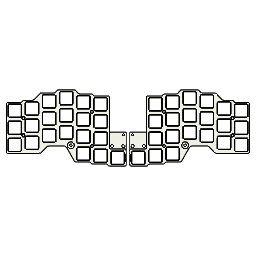
mriya-top-plate-v1.02 (Autodesk Fusion 360 design; units mm, degrees)
Autodesk Fusion 360 part; units mm, degrees
note: some values were not read from the file. Set by a fixed rule: which sketch regions a step uses.
sketch "mriya-top-plate" plane through (0, 0, 0) normal (0, 0, 1) x (1, 0, 0)
  arc A0 (-117.8, 77.3932) -> (-119.9, 79.4932) centre (-119.9, 77.3932) ccw
  line L0 (-132.4, 59.0932) -> (-132.4, 46.6932)
  line L1 (-114, 60.4932) -> (-114, 49.6932)
  arc A1 (-131.6, 78.8932) -> (-132.4, 78.0932) centre (-131.6, 78.0932) ccw
  line L2 (-131.6, 59.8932) -> (-119.2, 59.8932)
  circle A2 centre (-115.9, 63.5432) radius 1.45
  line L3 (-117.8, 58.3932) -> (-117.8, 47.5932)
  line L4 (-130.9, 60.4932) -> (-119.9, 60.4932)
  arc A3 (-131.6, 59.8932) -> (-132.4, 59.0932) centre (-131.6, 59.0932) ccw
  line L5 (-130.9, 79.4932) -> (-119.9, 79.4932)
  arc A4 (-119.2, 64.8932) -> (-118.4, 65.6932) centre (-119.2, 65.6932) ccw
  line L6 (-130.9, 64.2932) -> (-120.1, 64.2932)
  line L7 (-134.6, 79.4932) -> (-134.6, 26.2932) construction
  line L8 (-133, 77.3932) -> (-133, 66.3932)
  line L9 (-133.1, 81.1432) -> (-119.0284, 81.1432)
  line L10 (-117.8, 77.3932) -> (-117.8, 66.5932)
  line L11 (-131.6, 78.8932) -> (-119.2, 78.8932)
  arc A5 (-115.0716, 83.4432) -> (-116.5919, 82.8135) centre (-115.0716, 81.2933) ccw
  line L12 (-106.1426, 83.2932) -> (-115.0716, 83.2932) construction
  arc A6 (-115.0716, 83.2932) -> (-116.4858, 82.7074) centre (-115.0716, 81.2933) ccw construction
  arc A7 (-119.0284, 80.9932) -> (-117.6142, 81.579) centre (-119.0284, 82.9932) ccw construction
  arc A8 (-118.4, 59.0932) -> (-119.2, 59.8932) centre (-119.2, 59.0932) ccw
  arc A9 (-133, 66.3932) -> (-130.9, 64.2932) centre (-130.9, 66.3932) ccw
  line L13 (-133, 58.3932) -> (-133, 47.3932)
  line L14 (-113.4, 61.3932) -> (-113.4, 48.9932)
  arc A10 (-133.1, 80.9932) -> (-134.6, 79.4932) centre (-133.1, 79.4932) ccw construction
  arc A11 (-133.1, 81.1432) -> (-134.75, 79.4932) centre (-133.1, 79.4932) ccw
  line L15 (-74.6, 40.6932) -> (-62.2, 40.6932)
  line L16 (-73.9, 40.0932) -> (-62.9, 40.0932)
  line L17 (-73.9, 78.0932) -> (-62.9, 78.0932)
  arc A12 (-134.6, 26.2932) -> (-133.1, 24.7932) centre (-133.1, 26.2932) ccw construction
  arc A13 (-131.6, 40.8932) -> (-132.4, 40.0932) centre (-131.6, 40.0932) ccw
  arc A14 (-130.9, 41.4932) -> (-133, 39.3932) centre (-130.9, 39.3932) ccw
  arc A15 (-119.2, 26.8932) -> (-118.4, 27.6932) centre (-119.2, 27.6932) ccw
  line L18 (-73.9, 55.2932) -> (-62.9, 55.2932)
  line L19 (-74.6, 54.6932) -> (-62.2, 54.6932)
  arc A16 (-114, 30.6932) -> (-111.9, 28.5932) centre (-111.9, 30.6932) ccw
  line L20 (-113.4, 42.3932) -> (-113.4, 29.9932)
  line L21 (-130.9, 26.2932) -> (-119.9, 26.2932)
  line L22 (-59.6047, 16.0356) -> (-67.8823, 30.687)
  arc A17 (-119.9, 26.2932) -> (-117.8, 28.3932) centre (-119.9, 28.3932) ccw
  line L23 (-74.6, 92.6932) -> (-62.2, 92.6932)
  line L24 (-132.4, 40.0932) -> (-132.4, 27.6932)
  arc A18 (-113.4, 29.9932) -> (-112.6, 29.1932) centre (-112.6, 29.9932) ccw
  line L25 (-130.9, 41.4932) -> (-119.9, 41.4932)
  arc A19 (-118.4, 40.0932) -> (-119.2, 40.8932) centre (-119.2, 40.0932) ccw
  line L26 (-77.0716, 94.7932) -> (-59.7284, 94.7932) construction
  line L27 (-114, 41.4932) -> (-114, 30.6932)
  arc A20 (-132.4, 27.6932) -> (-131.6, 26.8932) centre (-131.6, 27.6932) ccw
  arc A21 (-133, 28.3932) -> (-130.9, 26.2932) centre (-130.9, 28.3932) ccw
  line L28 (-117.8, 39.3932) -> (-117.8, 28.3932)
  line L29 (-131.6, 40.8932) -> (-119.2, 40.8932)
  line L30 (-73.9, 59.0932) -> (-62.9, 59.0932)
  arc A22 (-117.8, 39.3932) -> (-119.9, 41.4932) centre (-119.9, 39.3932) ccw
  line L31 (-131.6, 26.8932) -> (-119.2, 26.8932)
  line L32 (-74.6, 78.6932) -> (-62.2, 78.6932)
  line L33 (-112.6, 29.1932) -> (-100.2, 29.1932)
  line L34 (-111.9, 66.5932) -> (-100.9, 66.5932)
  line L35 (-130.9, 45.2932) -> (-120.1, 45.2932)
  arc A23 (-133, 47.3932) -> (-130.9, 45.2932) centre (-130.9, 47.3932) ccw
  line L36 (-112.6, 62.1932) -> (-100.2, 62.1932)
  arc A24 (-120.1, 45.2932) -> (-117.8, 47.5932) centre (-120.1, 47.5932) ccw
  arc A25 (-119.2, 45.8932) -> (-118.4, 46.6932) centre (-119.2, 46.6932) ccw
  line L37 (-133.1, 24.7932) -> (-98.1426, 24.7932) construction
  line L38 (-131.6, 45.8932) -> (-119.2, 45.8932)
  arc A26 (-132.4, 46.6932) -> (-131.6, 45.8932) centre (-131.6, 46.6932) ccw
  line L39 (-111.7, 62.7932) -> (-100.9, 62.7932)
  line L40 (-104.1274, 84.2779) -> (-97.5918, 90.8135)
  circle A27 centre (-63.3, 33.4932) radius 1.4
  arc A28 (-114, 49.6932) -> (-111.9, 47.5932) centre (-111.9, 49.6932) ccw
  line L41 (-111.9, 47.5932) -> (-100.9, 47.5932)
  arc A29 (-111.7, 43.7932) -> (-114, 41.4932) centre (-111.7, 41.4932) ccw
  circle A30 centre (-63.3, 33.4932) radius 3.8
  line L42 (-133.1, 24.6432) -> (-98.1426, 24.6432)
  line L43 (-133, 39.3932) -> (-133, 28.3932)
  line L44 (-74.6, 73.6932) -> (-62.2, 73.6932)
  line L45 (-118.4, 40.0932) -> (-118.4, 27.6932)
  arc A31 (-113.4, 48.9932) -> (-112.6, 48.1932) centre (-112.6, 48.9932) ccw
  circle A32 centre (-115.9, 44.5432) radius 1.45
  line L46 (-74.6, 59.6932) -> (-62.2, 59.6932)
  line L47 (-112.6, 81.1932) -> (-100.2, 81.1932)
  line L48 (-134.75, 79.4932) -> (-134.75, 26.2932)
  line L49 (-118.4, 59.0932) -> (-118.4, 46.6932)
  line L50 (-111.7, 43.7932) -> (-100.9, 43.7932)
  arc A33 (-113.4, 67.9932) -> (-112.6, 67.1932) centre (-112.6, 67.9932) ccw
  arc A34 (-111.9, 81.7932) -> (-114, 79.6932) centre (-111.9, 79.6932) ccw
  arc A35 (-106.1426, 83.4432) -> (-104.1274, 84.2779) centre (-106.1426, 86.2932) ccw
  line L51 (-111.9, 81.7932) -> (-100.9, 81.7932)
  arc A36 (-114, 68.6932) -> (-111.9, 66.5932) centre (-111.9, 68.6932) ccw
  line L52 (-112.6, 43.1932) -> (-100.2, 43.1932)
  arc A37 (-111.7, 62.7932) -> (-114, 60.4932) centre (-111.7, 60.4932) ccw
  arc A38 (-112.6, 81.1932) -> (-113.4, 80.3932) centre (-112.6, 80.3932) ccw
  arc A39 (-106.1426, 83.2932) -> (-104.0213, 84.1719) centre (-106.1426, 86.2932) ccw construction
  line L53 (-114, 79.6932) -> (-114, 68.6932)
  line L54 (-112.6, 48.1932) -> (-100.2, 48.1932)
  line L55 (-112.6, 67.1932) -> (-100.2, 67.1932)
  line L56 (-111.9, 28.5932) -> (-100.9, 28.5932)
  line L57 (-113.4, 80.3932) -> (-113.4, 67.9932)
  arc A40 (-112.6, 62.1932) -> (-113.4, 61.3932) centre (-112.6, 61.3932) ccw
  line L58 (-106.1426, 83.4432) -> (-115.0716, 83.4432)
  line L59 (-104.0213, 84.1719) -> (-97.4858, 90.7074) construction
  arc A41 (-10.1, 30.7932) -> (-10.1, 34.1932) centre (-10.1, 32.4932) ccw construction
  line L60 (-36.6, 33.8932) -> (-24.2, 33.8932)
  arc A42 (-43.2, 17.1932) -> (-42.4, 17.9932) centre (-43.2, 17.9932) ccw
  line L61 (-36.6, 28.8932) -> (-24.2, 28.8932)
  line L62 (-35.9, 14.2932) -> (-24.9, 14.2932)
  arc A43 (-62.9, 40.0932) -> (-60.8, 42.1932) centre (-62.9, 42.1932) ccw
  line L63 (-55.6, 31.1932) -> (-43.2, 31.1932)
  arc A44 (-43.9, 35.5932) -> (-41.8, 37.6932) centre (-43.9, 37.6932) ccw
  arc A45 (-41.7203, 14.4013) -> (-43.0284, 14.9432) centre (-43.0284, 13.0933) ccw
  line L64 (-35.7, 33.2932) -> (-24.9, 33.2932)
  arc A46 (-56.4, 17.9932) -> (-55.6, 17.1932) centre (-55.6, 17.9932) ccw
  line L65 (-54.9, 16.5932) -> (-43.9, 16.5932)
  line L66 (-39.0716, 12.6432) -> (-24.0284, 12.6432)
  arc A47 (-43.2, 36.1932) -> (-42.4, 36.9932) centre (-43.2, 36.9932) ccw
  arc A48 (-41.8, 29.4932) -> (-44.1, 31.7932) centre (-44.1, 29.4932) ccw
  arc A49 (-41.6142, 14.5074) -> (-43.0284, 15.0932) centre (-43.0284, 13.0933) ccw construction
  arc A50 (-43.9, 16.5932) -> (-41.8, 18.6932) centre (-43.9, 18.6932) ccw
  arc A51 (-42.4, 30.3932) -> (-43.2, 31.1932) centre (-43.2, 30.3932) ccw
  line L67 (-35.9, 29.4932) -> (-24.9, 29.4932)
  line L68 (-36.6, 14.8932) -> (-24.2, 14.8932)
  line L69 (-21.4858, 11.079) -> (-22.6142, 12.2074) construction
  arc A52 (-4.4, 25.7932) -> (-5.2, 26.5932) centre (-5.2, 25.7932) ccw
  line L70 (-18.4, 25.7932) -> (-18.4, 13.3932)
  line L71 (-21.5919, 10.9729) -> (-22.7203, 12.1013)
  line L72 (-17.6, 26.5932) -> (-5.2, 26.5932)
  line L73 (-16.9, 27.1932) -> (-5.7, 27.1932)
  line L74 (-4, 25.4932) -> (-4, 13.6932)
  line L75 (-4.4, 25.7932) -> (-4.4, 13.3932)
  arc A53 (-21.5919, 10.9729) -> (-20.0716, 10.3432) centre (-20.0716, 12.4932) ccw
  line L76 (-2.75, 22.8932) -> (-2.75, 16.2932)
  arc A54 (-3.6, 10.3432) -> (-1.95, 11.9932) centre (-3.6, 11.9932) ccw
  arc A55 (-24.9, 14.2932) -> (-22.8, 16.3932) centre (-24.9, 16.3932) ccw
  line L77 (-17.6, 12.5932) -> (-5.2, 12.5932)
  circle A56 centre (-17.6, 32.4932) radius 1.7
  arc A57 (-22.7203, 12.1013) -> (-24.0284, 12.6432) centre (-24.0284, 10.7933) ccw
  line L78 (-19, 25.0932) -> (-19, 14.0932)
  line L79 (-2.1, 11.9932) -> (-2.1, 28.6932) construction
  arc A58 (-17.6, 26.5932) -> (-18.4, 25.7932) centre (-17.6, 25.7932) ccw
  circle A59 centre (-5.1, 45.1932) radius 1.1
  arc A60 (-5.2, 12.5932) -> (-4.4, 13.3932) centre (-5.2, 13.3932) ccw
  arc A61 (-5.7, 11.9932) -> (-4, 13.6932) centre (-5.7, 13.6932) ccw
  arc A62 (-3.6, 10.4932) -> (-2.1, 11.9932) centre (-3.6, 11.9932) ccw construction
  arc A63 (-12.7, 34.1932) -> (-12.7, 30.7932) centre (-12.7, 32.4932) ccw construction
  line L80 (-22.8, 27.3932) -> (-22.8, 16.3932)
  arc A64 (-19, 14.0932) -> (-16.9, 11.9932) centre (-16.9, 14.0932) ccw
  arc A65 (-36.6, 28.8932) -> (-37.4, 28.0932) centre (-36.6, 28.0932) ccw
  arc A66 (-37.4, 15.6932) -> (-36.6, 14.8932) centre (-36.6, 15.6932) ccw
  circle A67 centre (-39.9, 32.5432) radius 1.45
  arc A68 (-21.4858, 11.079) -> (-20.0716, 10.4932) centre (-20.0716, 12.4932) ccw construction
  line L81 (-23.4, 28.0932) -> (-23.4, 15.6932)
  line L82 (-3.6, 10.3432) -> (-20.0716, 10.3432)
  arc A69 (-24.2, 14.8932) -> (-23.4, 15.6932) centre (-24.2, 15.6932) ccw
  arc A70 (-16.9, 27.1932) -> (-19, 25.0932) centre (-16.9, 25.0932) ccw
  line L83 (-16.9, 11.9932) -> (-5.7, 11.9932)
  arc A71 (-23.4, 28.0932) -> (-24.2, 28.8932) centre (-24.2, 28.0932) ccw
  arc A72 (-22.8, 27.3932) -> (-24.9, 29.4932) centre (-24.9, 27.3932) ccw
  arc A73 (-2.1, 28.6932) -> (-2.9, 29.4932) centre (-2.9, 28.6932) ccw construction
  arc A74 (-18.4, 13.3932) -> (-17.6, 12.5932) centre (-17.6, 13.3932) ccw
  arc A75 (-4, 25.4932) -> (-5.7, 27.1932) centre (-5.7, 25.4932) ccw
  line L84 (-3.6, 10.4932) -> (-20.0716, 10.4932) construction
  line L85 (-1.95, 11.9932) -> (-1.95, 34.4932)
  arc A76 (-22.6142, 12.2074) -> (-24.0284, 12.7932) centre (-24.0284, 10.7933) ccw construction
  arc A77 (-22.8, 84.3932) -> (-24.9, 86.4932) centre (-24.9, 84.3932) ccw
  arc A78 (-37.4, 53.6932) -> (-36.6, 52.8932) centre (-36.6, 53.6932) ccw
  arc A79 (-1.95, 47.3932) -> (-2.75, 48.1932) centre (-2.75, 47.3932) ccw
  line L86 (-20.7, 49.1932) -> (-20.7, 87.3432)
  arc A80 (-35.9, 67.4932) -> (-38, 65.3932) centre (-35.9, 65.3932) ccw
  arc A81 (-35.9, 48.4932) -> (-38, 46.3932) centre (-35.9, 46.3932) ccw
  line L87 (-54.9, 50.7932) -> (-43.9, 50.7932)
  line L88 (-22.8, 84.3932) -> (-22.8, 73.3932)
  arc A82 (-60.8, 53.1932) -> (-62.9, 55.2932) centre (-62.9, 53.1932) ccw
  arc A83 (-24.9, 52.2932) -> (-22.8, 54.3932) centre (-24.9, 54.3932) ccw
  arc A84 (-42.4, 49.3932) -> (-43.2, 50.1932) centre (-43.2, 49.3932) ccw
  arc A85 (-41.8, 48.6932) -> (-43.9, 50.7932) centre (-43.9, 48.6932) ccw
  line L89 (-1.95, 29.4932) -> (-20.7, 29.4932)
  line L90 (-12.7, 34.1932) -> (-10.1, 34.1932) construction
  arc A86 (-24.9, 33.2932) -> (-22.8, 35.3932) centre (-24.9, 35.3932) ccw
  line L91 (-10.1, 30.7932) -> (-12.7, 30.7932) construction
  circle A87 centre (-11.4, 32.4932) radius 1.15 construction
  line L92 (-19.7, 29.4932) -> (-2.9, 29.4932) construction
  circle A88 centre (-5.1, 32.4932) radius 1.7
  arc A89 (-24.2, 33.8932) -> (-23.4, 34.6932) centre (-24.2, 34.6932) ccw
  arc A90 (-37.4, 34.6932) -> (-36.6, 33.8932) centre (-36.6, 34.6932) ccw
  arc A91 (-40.4858, 13.379) -> (-39.0716, 12.7932) centre (-39.0716, 14.7932) ccw construction
  arc A92 (-35.9, 29.4932) -> (-38, 27.3932) centre (-35.9, 27.3932) ccw
  arc A93 (-38, 35.5932) -> (-35.7, 33.2932) centre (-35.7, 35.5932) ccw
  arc A94 (-38, 16.3932) -> (-35.9, 14.2932) centre (-35.9, 16.3932) ccw
  line L93 (-37.4, 28.0932) -> (-37.4, 15.6932)
  arc A95 (-58.3142, 94.2074) -> (-59.7284, 94.7932) centre (-59.7284, 92.7932) ccw construction
  line L94 (-61.4, 72.8932) -> (-61.4, 60.4932)
  line L95 (-36.6, 66.8932) -> (-24.2, 66.8932)
  line L96 (-35.7, 71.2932) -> (-24.9, 71.2932)
  arc A96 (-54.8797, 90.9851) -> (-53.5716, 90.4432) centre (-53.5716, 92.2931) ccw
  line L97 (-54.9, 73.5932) -> (-43.9, 73.5932)
  arc A97 (-58.2081, 94.3135) -> (-59.7284, 94.9432) centre (-59.7284, 92.7932) ccw
  line L98 (-54.9, 88.7932) -> (-43.9, 88.7932)
  line L99 (-35.9, 52.2932) -> (-24.9, 52.2932)
  arc A98 (-54.9, 88.7932) -> (-57, 86.6932) centre (-54.9, 86.6932) ccw
  line L100 (-61.4, 91.8932) -> (-61.4, 79.4932)
  line L101 (-58.2081, 94.3135) -> (-54.8797, 90.9851)
  line L102 (-56.4, 87.3932) -> (-56.4, 74.9932)
  arc A99 (-61.4, 91.8932) -> (-62.2, 92.6932) centre (-62.2, 91.8932) ccw
  line L103 (-55.6, 88.1932) -> (-43.2, 88.1932)
  line L104 (-55.6, 74.1932) -> (-43.2, 74.1932)
  line L105 (-60.8, 72.1932) -> (-60.8, 61.1932)
  arc A100 (-57, 75.6932) -> (-54.9, 73.5932) centre (-54.9, 75.6932) ccw
  circle A101 centre (-39.9, 70.5432) radius 1.45
  arc A102 (-54.9858, 90.879) -> (-53.5716, 90.2932) centre (-53.5716, 92.2931) ccw construction
  arc A103 (-38, 73.5932) -> (-35.7, 71.2932) centre (-35.7, 73.5932) ccw
  arc A104 (-62.9, 78.0932) -> (-60.8, 80.1932) centre (-62.9, 80.1932) ccw
  line L106 (-36.7716, 88.1432) -> (-21.5, 88.1432)
  arc A105 (-56.4, 74.9932) -> (-55.6, 74.1932) centre (-55.6, 74.9932) ccw
  line L107 (-53.5716, 90.4432) -> (-40.7284, 90.4432)
  line L108 (-53.5716, 90.2932) -> (-40.7284, 90.2932) construction
  arc A106 (-62.2, 78.6932) -> (-61.4, 79.4932) centre (-62.2, 79.4932) ccw
  line L109 (-57, 86.6932) -> (-57, 75.6932)
  arc A107 (-60.8, 91.1932) -> (-62.9, 93.2932) centre (-62.9, 91.1932) ccw
  arc A108 (-39.3142, 89.7074) -> (-40.7284, 90.2932) centre (-40.7284, 88.2932) ccw construction
  arc A109 (-38.0797, 88.6851) -> (-36.7716, 88.1432) centre (-36.7716, 89.9932) ccw
  line L110 (-37.4, 85.0932) -> (-37.4, 72.6932)
  arc A110 (-55.6, 88.1932) -> (-56.4, 87.3932) centre (-55.6, 87.3932) ccw
  arc A111 (-60.8, 72.1932) -> (-62.9, 74.2932) centre (-62.9, 72.1932) ccw
  arc A112 (-61.4, 72.8932) -> (-62.2, 73.6932) centre (-62.2, 72.8932) ccw
  line L111 (-60.8, 91.1932) -> (-60.8, 80.1932)
  line L112 (-38.0797, 88.6851) -> (-39.2081, 89.8135)
  line L113 (-58.3142, 94.2074) -> (-54.9858, 90.879) construction
  line L114 (-38.1858, 88.579) -> (-39.3142, 89.7074) construction
  line L115 (-99.4, 42.3932) -> (-99.4, 29.9932)
  arc A113 (-81.2, 37.1932) -> (-80.4, 37.9932) centre (-81.2, 37.9932) ccw
  arc A114 (-75.4, 41.4932) -> (-74.6, 40.6932) centre (-74.6, 41.4932) ccw
  line L116 (-95.9152, 25.5658) -> (-89.6726, 31.8084)
  line L117 (-96.0213, 25.6719) -> (-89.7787, 31.9145) construction
  arc A115 (-76, 42.1932) -> (-73.9, 40.0932) centre (-73.9, 42.1932) ccw
  line L118 (-42.4, 49.3932) -> (-42.4, 36.9932)
  arc A116 (-94.4, 37.9932) -> (-93.6, 37.1932) centre (-93.6, 37.9932) ccw
  arc A117 (-67.7517, 30.7608) -> (-71.2344, 32.7932) centre (-71.2344, 28.793) ccw construction
  arc A118 (-67.8823, 30.687) -> (-71.2344, 32.6432) centre (-71.2344, 28.793) ccw
  line L119 (-98.8, 41.6932) -> (-98.8, 30.6932)
  arc A119 (-98.1426, 24.7932) -> (-96.0213, 25.6719) centre (-98.1426, 27.7931) ccw construction
  arc A120 (-87.6574, 32.7932) -> (-89.7787, 31.9145) centre (-87.6573, 29.7931) ccw construction
  arc A121 (-99.4, 42.3932) -> (-100.2, 43.1932) centre (-100.2, 42.3932) ccw
  arc A122 (-87.6574, 32.6432) -> (-89.6726, 31.8084) centre (-87.6573, 29.7931) ccw
  line L120 (-20.7, 29.4932) -> (-20.7, 49.1932)
  line L121 (-36.6, 52.8932) -> (-24.2, 52.8932)
  line L122 (-57, 48.6932) -> (-57, 37.6932)
  circle A123 centre (-5.1, 45.1932) radius 2.2 construction
  line L123 (-35.9, 86.4932) -> (-24.9, 86.4932)
  line L124 (-1.95, 47.3932) -> (-1.95, 34.4932)
  line L125 (-60.8, 53.1932) -> (-60.8, 42.1932)
  line L126 (-36.7716, 87.9932) -> (-21.5, 87.9932) construction
  line L127 (-23.4, 47.0932) -> (-23.4, 34.6932)
  line L128 (-36.6, 47.8932) -> (-24.2, 47.8932)
  line L129 (-35.9, 48.4932) -> (-24.9, 48.4932)
  line L130 (-36.6, 85.8932) -> (-24.2, 85.8932)
  line L131 (-41.8, 48.6932) -> (-41.8, 37.6932)
  line L132 (-37.4, 47.0932) -> (-37.4, 34.6932)
  line L133 (-36.6, 71.8932) -> (-24.2, 71.8932)
  line L134 (-56.4, 49.3932) -> (-56.4, 36.9932)
  line L135 (-22.8, 46.3932) -> (-22.8, 35.3932)
  line L136 (-38, 46.3932) -> (-38, 35.5932)
  line L137 (-20.7, 30.4932) -> (-20.7, 87.1932) construction
  line L138 (-35.9, 67.4932) -> (-24.9, 67.4932)
  line L139 (-61.4, 53.8932) -> (-61.4, 41.4932)
  line L140 (-95, 68.6932) -> (-95, 57.6932)
  line L141 (-75.4, 72.8932) -> (-75.4, 60.4932)
  line L142 (-79.8, 68.6932) -> (-79.8, 57.6932)
  line L143 (-80.4, 69.3932) -> (-80.4, 56.9932)
  arc A124 (-82.2284, 91.2932) -> (-80.8142, 91.879) centre (-82.2284, 93.2932) ccw construction
  arc A125 (-79.8, 68.6932) -> (-81.9, 70.7932) centre (-81.9, 68.6932) ccw
  line L144 (-76, 72.1932) -> (-76, 61.1932)
  line L145 (-94.4, 69.3932) -> (-94.4, 56.9932)
  arc A126 (-112.6, 43.1932) -> (-113.4, 42.3932) centre (-112.6, 42.3932) ccw
  arc A127 (-134.75, 26.2932) -> (-133.1, 24.6432) centre (-133.1, 26.2932) ccw
  line L146 (-76, 91.1932) -> (-76, 80.1932)
  arc A128 (-73.9, 93.2932) -> (-76, 91.1932) centre (-73.9, 91.1932) ccw
  arc A129 (-77.0716, 94.9432) -> (-78.5919, 94.3135) centre (-77.0716, 92.7933) ccw
  arc A130 (-76, 80.1932) -> (-73.9, 78.0932) centre (-73.9, 80.1932) ccw
  arc A131 (-92.9, 89.7932) -> (-95, 87.6932) centre (-92.9, 87.6932) ccw
  line L147 (-78.4858, 94.2074) -> (-80.8142, 91.879) construction
  arc A132 (-73.9, 74.2932) -> (-76, 72.1932) centre (-73.9, 72.1932) ccw
  arc A133 (-74.6, 73.6932) -> (-75.4, 72.8932) centre (-74.6, 72.8932) ccw
  line L148 (-78.5919, 94.3135) -> (-80.9203, 91.9851)
  line L149 (-79.8, 87.6932) -> (-79.8, 76.6932)
  arc A134 (-75.4, 79.4932) -> (-74.6, 78.6932) centre (-74.6, 79.4932) ccw
  line L150 (-59.4741, 16.1094) -> (-67.7517, 30.7608) construction
  line L151 (-80.4, 88.3932) -> (-80.4, 75.9932)
  line L152 (-75.4, 91.8932) -> (-75.4, 79.4932)
  arc A135 (-77.0716, 94.7932) -> (-78.4858, 94.2074) centre (-77.0716, 92.7933) ccw construction
  arc A136 (-94.4, 75.9932) -> (-93.6, 75.1932) centre (-93.6, 75.9932) ccw
  line L153 (-96.0716, 91.4432) -> (-82.2284, 91.4432)
  arc A137 (-100.2, 67.1932) -> (-99.4, 67.9932) centre (-100.2, 67.9932) ccw
  line L154 (-93.6, 89.1932) -> (-81.2, 89.1932)
  arc A138 (-100.9, 66.5932) -> (-98.8, 68.6932) centre (-100.9, 68.6932) ccw
  arc A139 (-96.0716, 91.2932) -> (-97.4858, 90.7074) centre (-96.0716, 89.2933) ccw construction
  line L155 (-99.4, 80.3932) -> (-99.4, 67.9932)
  arc A140 (-96.0716, 91.4432) -> (-97.5918, 90.8135) centre (-96.0716, 89.2933) ccw
  arc A141 (-92.9, 70.7932) -> (-95, 68.6932) centre (-92.9, 68.6932) ccw
  line L156 (-92.9, 89.7932) -> (-81.9, 89.7932)
  line L157 (-93.6, 70.1932) -> (-81.2, 70.1932)
  line L158 (-95, 87.6932) -> (-95, 76.6932)
  arc A142 (-99.4, 80.3932) -> (-100.2, 81.1932) centre (-100.2, 80.3932) ccw
  line L159 (-92.9, 70.7932) -> (-81.9, 70.7932)
  line L160 (-92.9, 74.5932) -> (-81.9, 74.5932)
  line L161 (-94.4, 88.3932) -> (-94.4, 75.9932)
  line L162 (-93.6, 75.1932) -> (-81.2, 75.1932)
  arc A143 (-93.6, 89.1932) -> (-94.4, 88.3932) centre (-93.6, 88.3932) ccw
  arc A144 (-98.8, 79.6932) -> (-100.9, 81.7932) centre (-100.9, 79.6932) ccw
  arc A145 (-93.6, 70.1932) -> (-94.4, 69.3932) centre (-93.6, 69.3932) ccw
  arc A146 (-80.4, 88.3932) -> (-81.2, 89.1932) centre (-81.2, 88.3932) ccw
  line L163 (-96.0716, 91.2932) -> (-82.2284, 91.2932) construction
  arc A147 (-95, 76.6932) -> (-92.9, 74.5932) centre (-92.9, 76.6932) ccw
  arc A148 (-79.8, 87.6932) -> (-81.9, 89.7932) centre (-81.9, 87.6932) ccw
  arc A149 (-82.2284, 91.4432) -> (-80.9203, 91.9851) centre (-82.2284, 93.2932) ccw
  line L164 (-98.8, 79.6932) -> (-98.8, 68.6932)
  arc A150 (-81.9, 74.5932) -> (-79.8, 76.6932) centre (-81.9, 76.6932) ccw
  arc A151 (-80.4, 69.3932) -> (-81.2, 70.1932) centre (-81.2, 69.3932) ccw
  arc A152 (-81.2, 75.1932) -> (-80.4, 75.9932) centre (-81.2, 75.9932) ccw
  arc A153 (-20.7, 30.4932) -> (-19.7, 29.4932) centre (-19.7, 30.4932) ccw construction
  line L165 (-54.9, 35.5932) -> (-43.9, 35.5932)
  line L166 (-43.0284, 15.0932) -> (-57.7328, 15.0932) construction
  line L167 (-55.6, 17.1932) -> (-43.2, 17.1932)
  line L168 (-55.6, 36.1932) -> (-43.2, 36.1932)
  line L169 (-77.0716, 94.9432) -> (-59.7284, 94.9432)
  arc A154 (-57, 18.6932) -> (-54.9, 16.5932) centre (-54.9, 18.6932) ccw
  line L170 (-73.9, 74.2932) -> (-62.9, 74.2932)
  line L171 (-57, 29.6932) -> (-57, 18.6932)
  line L172 (-73.9, 93.2932) -> (-62.9, 93.2932)
  arc A155 (-59.6047, 16.0356) -> (-57.7328, 14.9432) centre (-57.7328, 17.0932) ccw
  line L173 (-43.0284, 14.9432) -> (-57.7328, 14.9432)
  arc A156 (-40.5919, 13.2729) -> (-39.0716, 12.6432) centre (-39.0716, 14.7932) ccw
  line L174 (-38, 27.3932) -> (-38, 16.3932)
  line L175 (-41.8, 29.4932) -> (-41.8, 18.6932)
  line L176 (-56.4, 30.3932) -> (-56.4, 17.9932)
  line L177 (-40.5919, 13.2729) -> (-41.7203, 14.4013)
  arc A157 (-55.6, 31.1932) -> (-56.4, 30.3932) centre (-55.6, 30.3932) ccw
  arc A158 (-57, 37.6932) -> (-54.9, 35.5932) centre (-54.9, 37.6932) ccw
  arc A159 (-54.9, 31.7932) -> (-57, 29.6932) centre (-54.9, 29.6932) ccw
  arc A160 (-59.4741, 16.1094) -> (-57.7328, 15.0932) centre (-57.7328, 17.0932) ccw construction
  line L178 (-40.4858, 13.379) -> (-41.6142, 14.5074) construction
  arc A161 (-56.4, 36.9932) -> (-55.6, 36.1932) centre (-55.6, 36.9932) ccw
  line L179 (-54.9, 31.7932) -> (-44.1, 31.7932)
  line L180 (-42.4, 30.3932) -> (-42.4, 17.9932)
  arc A162 (-62.2, 40.6932) -> (-61.4, 41.4932) centre (-62.2, 41.4932) ccw
  arc A163 (-93.6, 51.1932) -> (-94.4, 50.3932) centre (-93.6, 50.3932) ccw
  line L181 (-93.6, 37.1932) -> (-81.2, 37.1932)
  arc A164 (-81.9, 36.5932) -> (-79.8, 38.6932) centre (-81.9, 38.6932) ccw
  arc A165 (-95, 57.6932) -> (-92.9, 55.5932) centre (-92.9, 57.6932) ccw
  arc A166 (-79.8, 49.6932) -> (-81.9, 51.7932) centre (-81.9, 49.6932) ccw
  arc A167 (-94.4, 56.9932) -> (-93.6, 56.1932) centre (-93.6, 56.9932) ccw
  arc A168 (-100.2, 29.1932) -> (-99.4, 29.9932) centre (-100.2, 29.9932) ccw
  arc A169 (-98.8, 41.6932) -> (-100.9, 43.7932) centre (-100.9, 41.6932) ccw
  arc A170 (-95, 38.6932) -> (-92.9, 36.5932) centre (-92.9, 38.6932) ccw
  arc A171 (-100.2, 48.1932) -> (-99.4, 48.9932) centre (-100.2, 48.9932) ccw
  arc A172 (-100.9, 47.5932) -> (-98.8, 49.6932) centre (-100.9, 49.6932) ccw
  line L182 (-92.9, 55.5932) -> (-81.9, 55.5932)
  arc A173 (-100.9, 28.5932) -> (-98.8, 30.6932) centre (-100.9, 30.6932) ccw
  line L183 (-87.6574, 32.7932) -> (-71.2344, 32.7932) construction
  arc A174 (-98.1426, 24.6432) -> (-95.9152, 25.5658) centre (-98.1426, 27.7931) ccw
  line L184 (-92.9, 36.5932) -> (-81.9, 36.5932)
  line L185 (-87.6574, 32.6432) -> (-71.2344, 32.6432)
  arc A175 (-76, 61.1932) -> (-73.9, 59.0932) centre (-73.9, 61.1932) ccw
  line L186 (-93.6, 51.1932) -> (-81.2, 51.1932)
  arc A176 (-92.9, 51.7932) -> (-95, 49.6932) centre (-92.9, 49.6932) ccw
  line L187 (-94.4, 50.3932) -> (-94.4, 37.9932)
  arc A177 (-75.4, 60.4932) -> (-74.6, 59.6932) centre (-74.6, 60.4932) ccw
  arc A178 (-73.9, 55.2932) -> (-76, 53.1932) centre (-73.9, 53.1932) ccw
  line L188 (-98.8, 60.6932) -> (-98.8, 49.6932)
  arc A179 (-80.4, 50.3932) -> (-81.2, 51.1932) centre (-81.2, 50.3932) ccw
  line L189 (-93.6, 56.1932) -> (-81.2, 56.1932)
  arc A180 (-81.2, 56.1932) -> (-80.4, 56.9932) centre (-81.2, 56.9932) ccw
  line L190 (-79.8, 49.6932) -> (-79.8, 38.6932)
  arc A181 (-81.9, 55.5932) -> (-79.8, 57.6932) centre (-81.9, 57.6932) ccw
  line L191 (-75.4, 53.8932) -> (-75.4, 41.4932)
  line L192 (-99.4, 61.3932) -> (-99.4, 48.9932)
  arc A182 (-98.8, 60.6932) -> (-100.9, 62.7932) centre (-100.9, 60.6932) ccw
  arc A183 (-74.6, 92.6932) -> (-75.4, 91.8932) centre (-74.6, 91.8932) ccw
  line L193 (-80.4, 50.3932) -> (-80.4, 37.9932)
  arc A184 (-74.6, 54.6932) -> (-75.4, 53.8932) centre (-74.6, 53.8932) ccw
  arc A185 (-99.4, 61.3932) -> (-100.2, 62.1932) centre (-100.2, 61.3932) ccw
  line L194 (-95, 49.6932) -> (-95, 38.6932)
  line L195 (-76, 53.1932) -> (-76, 42.1932)
  line L196 (-92.9, 51.7932) -> (-81.9, 51.7932)
  arc A186 (-20.7, 87.3432) -> (-21.5, 88.1432) centre (-21.5, 87.3432) ccw
  line L197 (-23.4, 66.0932) -> (-23.4, 53.6932)
  arc A187 (-23.4, 85.0932) -> (-24.2, 85.8932) centre (-24.2, 85.0932) ccw
  arc A188 (-20.7, 49.1932) -> (-19.7, 48.1932) centre (-19.7, 49.1932) ccw
  arc A189 (-22.8, 65.3932) -> (-24.9, 67.4932) centre (-24.9, 65.3932) ccw
  arc A190 (-24.9, 71.2932) -> (-22.8, 73.3932) centre (-24.9, 73.3932) ccw
  line L198 (-39.0716, 12.7932) -> (-24.0284, 12.7932) construction
  arc A191 (-24.2, 71.8932) -> (-23.4, 72.6932) centre (-24.2, 72.6932) ccw
  arc A192 (-23.4, 47.0932) -> (-24.2, 47.8932) centre (-24.2, 47.0932) ccw
  line L199 (-23.4, 85.0932) -> (-23.4, 72.6932)
  arc A193 (-22.8, 46.3932) -> (-24.9, 48.4932) centre (-24.9, 46.3932) ccw
  line L200 (-22.8, 65.3932) -> (-22.8, 54.3932)
  line L201 (-19.7, 48.1932) -> (-2.75, 48.1932)
  arc A194 (-20.7, 87.1932) -> (-21.5, 87.9932) centre (-21.5, 87.1932) ccw construction
  arc A195 (-24.2, 52.8932) -> (-23.4, 53.6932) centre (-24.2, 53.6932) ccw
  arc A196 (-23.4, 66.0932) -> (-24.2, 66.8932) centre (-24.2, 66.0932) ccw
  line L202 (-42.4, 68.3932) -> (-42.4, 55.9932)
  arc A197 (-36.6, 85.8932) -> (-37.4, 85.0932) centre (-36.6, 85.0932) ccw
  arc A198 (-43.2, 74.1932) -> (-42.4, 74.9932) centre (-43.2, 74.9932) ccw
  arc A199 (-38.1858, 88.579) -> (-36.7716, 87.9932) centre (-36.7716, 89.9932) ccw construction
  arc A200 (-61.4, 53.8932) -> (-62.2, 54.6932) centre (-62.2, 53.8932) ccw
  arc A201 (-37.4, 72.6932) -> (-36.6, 71.8932) centre (-36.6, 72.6932) ccw
  arc A202 (-36.6, 47.8932) -> (-37.4, 47.0932) centre (-36.6, 47.0932) ccw
  arc A203 (-43.9, 73.5932) -> (-41.8, 75.6932) centre (-43.9, 75.6932) ccw
  arc A204 (-35.9, 86.4932) -> (-38, 84.3932) centre (-35.9, 84.3932) ccw
  arc A205 (-39.2081, 89.8135) -> (-40.7284, 90.4432) centre (-40.7284, 88.2932) ccw
  line L203 (-41.8, 86.6932) -> (-41.8, 75.6932)
  line L204 (-37.4, 66.0932) -> (-37.4, 53.6932)
  arc A206 (-54.9, 50.7932) -> (-57, 48.6932) centre (-54.9, 48.6932) ccw
  arc A207 (-41.8, 86.6932) -> (-43.9, 88.7932) centre (-43.9, 86.6932) ccw
  line L205 (-57, 67.6932) -> (-57, 56.6932)
  line L206 (-38, 84.3932) -> (-38, 73.5932)
  arc A208 (-57, 56.6932) -> (-54.9, 54.5932) centre (-54.9, 56.6932) ccw
  arc A209 (-42.4, 87.3932) -> (-43.2, 88.1932) centre (-43.2, 87.3932) ccw
  line L207 (-42.4, 87.3932) -> (-42.4, 74.9932)
  arc A210 (-55.6, 69.1932) -> (-56.4, 68.3932) centre (-55.6, 68.3932) ccw
  arc A211 (-54.9, 69.7932) -> (-57, 67.6932) centre (-54.9, 67.6932) ccw
  line L208 (-54.9, 69.7932) -> (-44.1, 69.7932)
  line L209 (-55.6, 55.1932) -> (-43.2, 55.1932)
  line L210 (-55.6, 50.1932) -> (-43.2, 50.1932)
  arc A212 (-62.2, 59.6932) -> (-61.4, 60.4932) centre (-62.2, 60.4932) ccw
  line L211 (-41.8, 67.4932) -> (-41.8, 56.6932)
  arc A213 (-56.4, 55.9932) -> (-55.6, 55.1932) centre (-55.6, 55.9932) ccw
  arc A214 (-41.8, 67.4932) -> (-44.1, 69.7932) centre (-44.1, 67.4932) ccw
  arc A215 (-43.9, 54.5932) -> (-41.8, 56.6932) centre (-43.9, 56.6932) ccw
  arc A216 (-43.2, 55.1932) -> (-42.4, 55.9932) centre (-43.2, 55.9932) ccw
  line L212 (-56.4, 68.3932) -> (-56.4, 55.9932)
  arc A217 (-55.6, 50.1932) -> (-56.4, 49.3932) centre (-55.6, 49.3932) ccw
  arc A218 (-62.9, 59.0932) -> (-60.8, 61.1932) centre (-62.9, 61.1932) ccw
  arc A219 (-36.6, 66.8932) -> (-37.4, 66.0932) centre (-36.6, 66.0932) ccw
  line L213 (-55.6, 69.1932) -> (-43.2, 69.1932)
  arc A220 (-42.4, 68.3932) -> (-43.2, 69.1932) centre (-43.2, 68.3932) ccw
  arc A221 (-38, 54.3932) -> (-35.9, 52.2932) centre (-35.9, 54.3932) ccw
  line L214 (-54.9, 54.5932) -> (-43.9, 54.5932)
  line L215 (-38, 65.3932) -> (-38, 54.3932)
  arc A222 (-130.9, 60.4932) -> (-133, 58.3932) centre (-130.9, 58.3932) ccw
  arc A223 (-120.1, 64.2932) -> (-117.8, 66.5932) centre (-120.1, 66.5932) ccw
  line L216 (-117.7203, 81.6851) -> (-116.5919, 82.8135)
  arc A224 (-119.0284, 81.1432) -> (-117.7203, 81.6851) centre (-119.0284, 82.9932) ccw
  line L217 (-131.6, 64.8932) -> (-119.2, 64.8932)
  line L218 (-132.4, 78.0932) -> (-132.4, 65.6932)
  line L219 (-118.4, 78.0932) -> (-118.4, 65.6932)
  line L220 (-117.6142, 81.579) -> (-116.4858, 82.7074) construction
  arc A225 (-117.8, 58.3932) -> (-119.9, 60.4932) centre (-119.9, 58.3932) ccw
  line L221 (-133.1, 80.9932) -> (-119.0284, 80.9932) construction
  arc A226 (-118.4, 78.0932) -> (-119.2, 78.8932) centre (-119.2, 78.0932) ccw
  arc A227 (-130.9, 79.4932) -> (-133, 77.3932) centre (-130.9, 77.3932) ccw
  arc A228 (-132.4, 65.6932) -> (-131.6, 64.8932) centre (-131.6, 65.6932) ccw
  arc A229 (-1.95, 23.6932) -> (-2.75, 22.8932) centre (-1.95, 22.8932) ccw
  arc A230 (-2.75, 16.2932) -> (-1.95, 15.4932) centre (-1.95, 16.2932) ccw
  dimension "d1" = 2.9
  dimension "d2" = 2.9
  dimension "d3" = 2.8
  dimension "d4" = 2.9
  dimension "d5" = 2.9
  dimension "d6" = 3.4
  dimension "d7" = 3.4
  dimension "d8" = 7.6
  dimension "d9" = 2.3
  dimension "d10" = 2.2
  dimension "d11" = 4.4
  constraint tangent L114 A199
  constraint tangent A108 L114
  constraint tangent A102 L108
  constraint tangent A95 L113
  constraint tangent L26 A135
  constraint tangent A124 L147
  constraint tangent A139 L163
  constraint tangent A7 L220
  constraint tangent A10 L221
  constraint tangent L7 A12
  constraint tangent L37 A119
  constraint tangent L117 A120
  constraint tangent A117 L183
  constraint tangent L150 A160
  constraint tangent A49 L166
  constraint tangent A91 L178
  constraint tangent A76 L198
  constraint tangent L69 A68
  constraint tangent A62 L84
  constraint tangent L79 A62
  constraint perpendicular L79 L126
  constraint perpendicular L126 L137
  constraint perpendicular L79 L92
  constraint tangent A1 L218
  constraint tangent L11 A226
  constraint tangent A4 L219
  constraint tangent L217 A228
  constraint tangent L2 A3
  constraint tangent L2 A8
  constraint tangent A25 L49
  constraint tangent L38 A26
  constraint tangent A13 L29
  constraint tangent A19 L29
  constraint tangent A15 L45
  constraint tangent A20 L31
  constraint tangent L20 A18
  constraint tangent L33 A168
  constraint tangent L115 A121
  constraint tangent L52 A126
  constraint tangent L54 A171
  constraint tangent A31 L54
  constraint tangent L14 A40
  constraint tangent L36 A185
  constraint tangent A33 L55
  constraint tangent L55 A137
  constraint tangent A137 L155
  constraint tangent L155 A142
  constraint tangent L47 A38
  constraint tangent L161 A143
  constraint tangent L154 A146
  constraint tangent L151 A152
  constraint tangent A136 L162
  constraint tangent L157 A145
  constraint tangent L157 A151
  constraint tangent L143 A180
  constraint tangent A167 L189
  constraint tangent A163 L186
  constraint tangent A116 L187
  constraint tangent A116 L181
  constraint tangent A113 L181
  constraint tangent A179 L193
  constraint tangent A114 L191
  constraint tangent L15 A114
  constraint tangent L191 A184
  constraint tangent L19 A200
  constraint tangent L139 A162
  constraint tangent L46 A212
  constraint tangent L46 A177
  constraint tangent L141 A133
  constraint tangent L44 A112
  constraint tangent L32 A106
  constraint tangent L32 A134
  constraint tangent L152 A183
  constraint tangent L23 A99
  constraint tangent L102 A110
  constraint tangent L102 A105
  constraint tangent L104 A105
  constraint tangent L104 A198
  constraint tangent A198 L207
  constraint tangent A209 L207
  constraint tangent L103 A209
  constraint tangent L213 A220
  constraint tangent A210 L213
  constraint tangent A213 L212
  constraint tangent L209 A216
  constraint tangent A84 L210
  constraint tangent L210 A217
  constraint tangent L134 A217
  constraint tangent L134 A161
  constraint tangent L168 A161
  constraint tangent A47 L168
  constraint tangent A47 L118
  constraint tangent L63 A51
  constraint tangent L63 A157
  constraint tangent L176 A157
  constraint tangent A46 L176
  constraint tangent A42 L167
  constraint tangent A66 L93
  constraint tangent L68 A69
  constraint tangent L81 A71
  constraint tangent L61 A71
  constraint tangent L61 A65
  constraint tangent A65 L93
  constraint tangent L70 A74
  constraint tangent L77 A74
  constraint tangent L77 A60
  constraint tangent L75 A60
  constraint tangent A52 L75
  constraint tangent A52 L72
  constraint tangent L72 A58
  constraint tangent L70 A58
  constraint tangent L60 A89
  constraint tangent A89 L127
  constraint tangent L60 A90
  constraint tangent L132 A202
  constraint tangent L128 A192
  constraint tangent L121 A195
  constraint tangent L197 A195
  constraint tangent A78 L121
  constraint tangent L204 A219
  constraint tangent L95 A196
  constraint tangent L133 A191
  constraint tangent A191 L199
  constraint tangent L133 A201
  constraint tangent L110 A197
  constraint tangent L130 A187
  constraint tangent L137 A194
  constraint tangent L126 A194
  constraint tangent L59 A139
  constraint tangent L12 A6
  constraint tangent A39 L59
  constraint tangent L12 A39
  constraint horizontal L92
  constraint tangent L137 A153
  constraint tangent L92 A153
  constraint tangent A73 L92
  constraint tangent L79 A73
  constraint tangent A188 L201
  constraint tangent L86 A188
  constraint concentric A27 A30
  constraint tangent L120 A188
  constraint concentric A117 A118
  constraint concentric A120 A122
  constraint concentric A119 A174
  constraint concentric A12 A127
  constraint concentric A10 A11
  constraint concentric A7 A224
  constraint concentric A5 A6
  constraint concentric A35 A39
  constraint concentric A139 A140
  constraint concentric A124 A149
  constraint concentric A129 A135
  constraint concentric A95 A97
  constraint concentric A96 A102
  constraint concentric A108 A205
  constraint concentric A109 A199
  constraint concentric A54 A62
  constraint concentric A53 A68
  constraint concentric A57 A76
  constraint concentric A91 A156
  constraint concentric A45 A49
  constraint concentric A155 A160
  constraint tangent L116 A122
  constraint tangent A118 L185
  constraint tangent A11 L48
  constraint tangent L66 A57
  constraint tangent L42 A174
  constraint tangent L40 A140
  constraint tangent L42 A127
  constraint tangent L48 A127
  constraint tangent L9 A11
  constraint tangent L216 A224
  constraint tangent A54 L85
  constraint tangent A109 L112
  constraint tangent A5 L58
  constraint tangent L112 A205
  constraint tangent A35 L58
  constraint tangent L40 A35
  constraint tangent L153 A140
  constraint tangent A45 L173
  constraint tangent L148 A149
  constraint tangent A129 L169
  constraint tangent A97 L101
  constraint tangent A156 L177
  constraint tangent A96 L107
  constraint tangent L71 A53
  constraint tangent A54 L82
  constraint tangent L5 A227
  constraint tangent L8 A227
  constraint tangent A0 L5
  constraint tangent A0 L10
  constraint tangent L8 A9
  constraint tangent L6 A9
  constraint tangent L34 A138
  constraint tangent A138 L164
  constraint tangent A34 L51
  constraint tangent A34 L53
  constraint tangent L51 A144
  constraint tangent A144 L164
  constraint tangent A36 L53
  constraint tangent L34 A36
  constraint tangent L160 A150
  constraint tangent L149 A150
  constraint tangent A131 L156
  constraint tangent A131 L158
  constraint tangent L156 A148
  constraint tangent L149 A148
  constraint tangent L158 A147
  constraint tangent L160 A147
  constraint tangent L17 A104
  constraint tangent A104 L111
  constraint tangent A128 L172
  constraint tangent L146 A128
  constraint tangent A107 L172
  constraint tangent A107 L111
  constraint tangent L146 A130
  constraint tangent L17 A130
  constraint tangent L97 A203
  constraint tangent A203 L203
  constraint tangent L98 A98
  constraint tangent A98 L109
  constraint tangent L98 A207
  constraint tangent L203 A207
  constraint tangent A100 L109
  constraint tangent L97 A100
  constraint tangent L96 A190
  constraint tangent L88 A190
  constraint tangent L123 A204
  constraint tangent A204 L206
  constraint tangent A77 L123
  constraint tangent A77 L88
  constraint tangent L4 A222
  constraint tangent L13 A222
  constraint tangent L4 A225
  constraint tangent L3 A225
  constraint tangent L13 A23
  constraint tangent L35 A23
  constraint tangent L41 A172
  constraint tangent A172 L188
  constraint tangent L39 A182
  constraint tangent L188 A182
  constraint tangent L1 A28
  constraint tangent A28 L41
  constraint tangent L182 A181
  constraint tangent L142 A181
  constraint tangent A141 L159
  constraint tangent L140 A141
  constraint tangent A125 L159
  constraint tangent L142 A125
  constraint tangent L140 A165
  constraint tangent A165 L182
  constraint tangent L30 A218
  constraint tangent L105 A218
  constraint tangent A132 L170
  constraint tangent L144 A132
  constraint tangent A111 L170
  constraint tangent L105 A111
  constraint tangent L144 A175
  constraint tangent L30 A175
  constraint tangent A215 L214
  constraint tangent L211 A215
  constraint tangent A211 L208
  constraint tangent L205 A211
  constraint tangent L205 A208
  constraint tangent A208 L214
  constraint tangent A83 L99
  constraint tangent A83 L200
  constraint tangent A80 L138
  constraint tangent A80 L215
  constraint tangent L138 A189
  constraint tangent A189 L200
  constraint tangent A221 L215
  constraint tangent L99 A221
  constraint tangent L21 A17
  constraint tangent A17 L28
  constraint tangent A14 L25
  constraint tangent A14 L43
  constraint tangent L25 A22
  constraint tangent L28 A22
  constraint tangent A21 L43
  constraint tangent L21 A21
  constraint tangent L56 A173
  constraint tangent L119 A173
  constraint tangent L50 A169
  constraint tangent L119 A169
  constraint tangent A16 L27
  constraint tangent A16 L56
  constraint tangent A164 L184
  constraint tangent A164 L190
  constraint tangent A176 L196
  constraint tangent A176 L194
  constraint tangent A166 L196
  constraint tangent A166 L190
  constraint tangent A170 L194
  constraint tangent A170 L184
  constraint tangent L16 A43
  constraint tangent A43 L125
  constraint tangent L18 A178
  constraint tangent A178 L195
  constraint tangent L18 A82
  constraint tangent A82 L125
  constraint tangent A115 L195
  constraint tangent L16 A115
  constraint tangent A44 L165
  constraint tangent A44 L131
  constraint tangent L87 A206
  constraint tangent L122 A206
  constraint tangent L87 A85
  constraint tangent A85 L131
  constraint tangent L122 A158
  constraint tangent L165 A158
  constraint tangent L64 A86
  constraint tangent A86 L135
  constraint tangent A81 L129
  constraint tangent A81 L136
  constraint tangent L129 A193
  constraint tangent L135 A193
  constraint tangent L65 A50
  constraint tangent A50 L175
  constraint tangent A159 L179
  constraint tangent L171 A159
  constraint tangent A154 L171
  constraint tangent L65 A154
  constraint tangent L62 A55
  constraint tangent A55 L80
  constraint tangent L67 A92
  constraint tangent A92 L174
  constraint tangent L67 A72
  constraint tangent L80 A72
  constraint tangent A94 L174
  constraint tangent L62 A94
  constraint tangent L73 A70
  constraint tangent L78 A70
  constraint tangent L78 A64
  constraint tangent A64 L83
  constraint tangent L73 A75
  constraint tangent L74 A75
  constraint tangent L74 A61
  constraint tangent A61 L83
  constraint tangent A79 L201
  constraint tangent L85 A79
  constraint tangent L106 A186
  constraint tangent L86 A186
  constraint tangent A41 L90
  constraint tangent A63 L91
  constraint tangent L39 A37
  constraint tangent L1 A37
  constraint tangent L6 A223
  constraint tangent L10 A223
  constraint tangent L3 A24
  constraint tangent L35 A24
  constraint tangent A29 L50
  constraint tangent L27 A29
  constraint tangent L208 A214
  constraint tangent L211 A214
  constraint tangent A103 L206
  constraint tangent L96 A103
  constraint tangent A48 L179
  constraint tangent A48 L175
  constraint tangent A93 L136
  constraint tangent L64 A93
  constraint concentric A59 A123
  constraint coincident L89.start L85
  constraint tangent L76 A229
  constraint tangent L76 A230
  measures "d1" diameter of A2
  measures "d2" diameter of A32
  measures "d3" diameter of A27
  measures "d4" diameter of A67
  measures "d5" diameter of A101
  measures "d6" diameter of A88
  measures "d7" diameter of A56
  measures "d8" diameter of A30
  measures "d9" diameter of A87
  measures "d10" diameter of A59
  measures "d11" diameter of A123
extrude "Extrude1" add sketch "mriya-top-plate" along normal blind 1.5 contours A0 L5 L6 L8 L10 A9 A223 A227 | L1 L39 A28 L41 A37 A172 L188 A182 | A2 | L3 L4 L13 L35 A23 A24 A222 A225 | L76 L85 A229 A230 | L85 A79 L89 L120 L124 A188 L201 | L16 L18 A43 A82 A115 L125 A178 L195 | L17 A104 A107 L111 L146 A128 A130 L172 | A14 L21 A17 L25 A21 L28 A22 L43 | A16 L27 A29 L50 L56 L119 A169 A173 | L30 L105 A111 L144 A132 L170 A175 A218 | L34 A34 L51 A36 L53 A138 A144 L164 | A30 | A32 | L62 L67 A55 L80 A72 A92 A94 L174 | A44 L87 A85 L122 L131 L165 A158 A206 | L64 A81 A86 A93 L129 L135 L136 A193 | L65 A48 A50 A154 L171 L175 A159 L179 | L73 L74 L78 A61 A64 A70 L83 A75 | A67 | A77 L88 L96 A103 L123 A190 A204 L206 | A80 A83 L99 L138 A189 L200 A221 L215 | L97 L98 A98 A100 L109 A203 L203 A207 | A101 | L140 L142 A125 A141 L159 A165 L182 A181 | A131 L149 L156 L158 L160 A147 A148 A150 | A164 A166 A170 L184 A176 L190 L194 L196 | L205 A208 A211 L208 L211 A214 A215 L214 makes body 1 at (-114.9406, 45.6304, 1) makes body 2 at (-118.2, 51.1265, 0) makes body 3 at (-113.6, 37.9599, 0) makes body 4 at (-61.2, 87.5265, 0) makes body 5 at (-42.2, 25.9599, 0) makes body 6 at (-32.1667, 71.6932, 0) makes body 7 at (-13.2333, 12.3932, 0) makes body 8 at (-23.2, 23.7265, 0) makes body 9 at (-42.2, 83.0265, 0) makes body 10 at (-63.7804, 36.4462, 0) makes body 11 at (-89.2333, 74.9932, 0) makes body 12 at (-113.6, 56.9599, 0) makes body 13 at (-127.2333, 41.0932, 0) makes body 14 at (-116.8594, 62.456, 1) makes body 15 at (-38.7442, 71.4187, 1) makes body 16 at (-118.2, 70.1265, 0) makes body 17 at (-94.6, 46.0265, 0) makes body 18 at (-61.2, 68.5265, 0) makes body 19 at (-42.2, 45.0265, 0) makes body 20 at (-23.2, 61.7265, 0) makes body 21 at (-14.2767, 42.3793, 0) makes body 22 at (-32.1667, 33.6932, 0) makes body 23 at (-42.2, 63.9599, 0) makes body 24 at (-61.2, 49.5265, 0) makes body 25 at (-80.2, 65.0265, 0) makes body 26 at (-113.6, 76.0265, 0) makes body 27 at (-39.3036, 33.8649, 1) makes body 28 at (-1.95, 18.2265, 0.5)
extrude "Extrude2" add sketch "mriya-top-plate" along normal blind 5 contours L9 A5 A11 L22 L40 L42 L48 A35 L58 A45 L66 L71 A53 L76 A54 A57 L82 L85 L86 L89 A96 A97 L101 L106 L107 A109 L112 L116 A118 A122 L120 A127 A129 L148 L153 A140 A149 L169 A155 L173 A156 L177 A174 L185 A186 A205 L216 A224 A229 A230 bodies 1 2 3 4 5 6 7 8 9 10 11 12 13 14 15 16 17 18 19 20 21 22 23 24 25 26 27 28
fillet "Fillet2" radius 1.65 2 edges at (-1.95, 29.4932, 3.25) (-20.7, 29.4932, 3.25) on bodies 1
fillet "Fillet4" radius 0.6 2 edges at (-1.95, 23.6932, 3.25) (-1.95, 15.4932, 3.25) on bodies 1
chamfer "Chamfer1" distance 0.4 angle 45 4 edges at (-41.2519, 33.0675, 5) (-41.2519, 71.0675, 5) (-117.2519, 64.0675, 5) (-117.2519, 45.0675, 5) on bodies 1
mirror "Mirror1" about plane through (0, 0, 0) normal (1, 0, 0) of bodies 1 makes body 29
named bodies: "right", "left"
